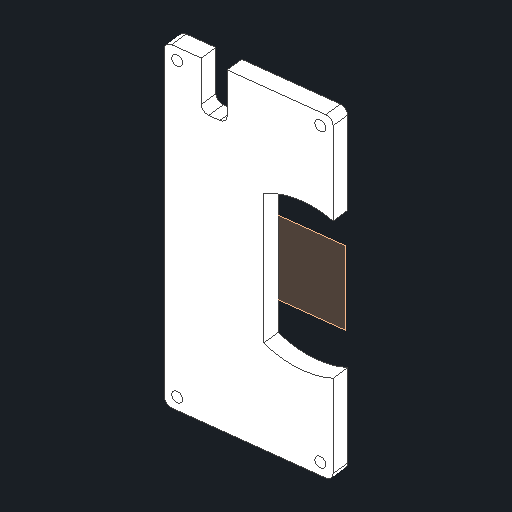
# Autodesk Inventor part: TAPA_CAMARA_2
Saved by Autodesk Inventor 2024.3 (Build 283343000, 343)
## iProperties
Created: 2024-07-21
Part Number: TAPA_CAMARA_2
Material: Generic
Document SubType Name: Modeling
Designer: Niler
Density: 1 g/cm^3
Appearance: Default
Author: Niler
Autodesk Inventor part; units mm, degrees
ref_plane "YZ Plane" through (0, 0, 0) normal (1, 0, 0) x (0, 1, 0)
ref_plane "XZ Plane" through (0, 0, 0) normal (0, 1, 0) x (-1, 0, 0)
ref_plane "XY Plane" through (0, 0, 0) normal (0, 0, 1) x (1, 0, 0)
ref_plane "Work Plane1" through (-27.4782, 47.3, -1.2107) normal (0.118263, 0, 0.9929823) x (0, -1, 0)
sketch "Sketch1" plane through (-27.4782, 47.3, -1.2107) normal (0.118263, 0, 0.9929823) x (0, -1, 0)
  line L0 (0, 33.4421) -> (0, -8.2516) projected
  line L1 (2, -10.2376) -> (92.6, -10.2376) projected
  line L2 (94.6, -8.2516) -> (94.6, 33.4421) projected
  line L3 (92.6, 35.428) -> (2, 35.428) projected
  line L4 (7, -3.2867) -> (7, 28.4771) projected
  line L5 (7, 28.4771) -> (87.6, 28.4771) projected
  line L6 (87.6, 28.4771) -> (87.6, -3.2867) projected
  line L7 (87.6, -3.2867) -> (7, -3.2867) projected
  ellipse E0 centre (2, 33.4421) end of major axis (4, 33.4421) minor radius 1.986 (2, 35.428) -> (0, 33.4421) ccw projected
  ellipse E1 centre (2, -8.2516) end of major axis (0, -8.2516) minor radius 1.986 (0, -8.2516) -> (2, -10.2376) ccw projected
  ellipse E2 centre (92.6, -8.2516) end of major axis (90.6, -8.2516) minor radius 1.986 (92.6, -10.2376) -> (94.6, -8.2516) ccw projected
  ellipse E3 centre (92.6, 33.4421) end of major axis (94.6, 33.4421) minor radius 1.986 (94.6, 33.4421) -> (92.6, 35.428) ccw projected
  ellipse E4 centre (91.1, -6.7621) end of major axis (92.6, -6.7621) minor radius 1.4895 projected
  ellipse E5 centre (3.5, -6.7621) end of major axis (5, -6.7621) minor radius 1.4895 projected
  ellipse E6 centre (91.1, 31.9526) end of major axis (92.6, 31.9526) minor radius 1.4895 projected
  ellipse E7 centre (3.5, 31.9526) end of major axis (5, 31.9526) minor radius 1.4895 projected
  point P0 (47.3, 27.1422)
  constraints: 4 other
extrude "Extrusion1" add sketch "Sketch1" along normal blind 5 contours E0 L3 E3 L2 E2 L1 E1 L0 | L4 L5 L6 L7
sketch "Sketch2" plane through (-26.8869, 47.3, 3.7542) normal (0.118263, 0, 0.9929823) x (0.9929823, 0, -0.118263)
  line L0 (16.6422, -25.3) -> (37.6422, -25.3)
  line L1 (37.6422, -25.3) -> (37.6422, -69.3)
  line L2 (37.6422, -69.3) -> (16.6422, -69.3)
  line L3 (16.6422, -69.3) -> (16.6422, -25.3)
  line L4 (16.6422, -25.3) -> (37.6422, -69.3) construction
  line L5 (37.6422, -25.3) -> (16.6422, -69.3) construction
  line L6 (37.6422, -27.8) -> (16.6422, -27.8)
  arc A0 (37.6422, -27.8) -> (16.6422, -27.8) centre (27.1422, -48.6) ccw
  line L7 (33.4421, 0) -> (-8.2516, 0) projected
  arc A1 (-8.2516, 0) -> (-10.2376, -2) centre (2, -2) ccw projected
  line L8 (-10.2376, -2) -> (-10.2376, -92.6) projected
  arc A2 (-10.2376, -92.6) -> (-8.2516, -94.6) centre (2, -92.6) ccw projected
  line L9 (-8.2516, -94.6) -> (33.4421, -94.6) projected
  arc A3 (33.4421, -94.6) -> (35.428, -92.6) centre (45.9099, -92.6) ccw projected
  line L10 (35.428, -92.6) -> (35.428, -2) projected
  arc A4 (35.428, -2) -> (33.4421, 0) centre (45.9099, -2) ccw projected
  circle A5 centre (44.4099, -3.5) radius 1.5 projected
  circle A6 centre (44.4099, -91.1) radius 1.5 projected
  circle A7 centre (3.5, -3.5) radius 1.5 projected
  circle A8 centre (3.5, -91.1) radius 1.5 projected
  line L11 (35.428, -47.3) -> (-10.2376, -47.3)
  line L12 (-10.2376, -2) -> (-10.2376, -92.6) projected
  arc A9 (16.6422, -66.8) -> (37.6422, -66.8) centre (27.1422, -46) ccw
  point P0 (27.1422, -47.3)
  point P1 (27.1422, -25.3)
  point P2 (16.6422, -66.8)
  point P3 (37.6422, -66.8)
  dimension "d2" = 21
  dimension "d3" = 44
  dimension "d4" = 2.5
  constraints: 16 end point, 5 midpoint, 5 point on circle, 3 symmetric about line, 2 centre point, 2 parallel, 2 perpendicular, 2 point on line, 1 horizontal, 5 other
  measures "d2" distance of L1.end L2.end
  measures "d3" distance of L0.end L1.end
  measures "d4" distance between parallel lines of L0 L6
extrude "Extrusion2" cut sketch "Sketch2" against normal through all contours A0 L10 L6 | L6 L10 L11 L3 | A0 L6 L10 | L11 L10 A9 L3 | L6 L1 A9 L10
sketch "Sketch3" plane through (-27.4782, 47.3, -1.2107) normal (-0.118263, 0, -0.9929823) x (-0.9929823, 0, 0.118263)
  arc A0 (-35.428, -67.7769) -> (-16.6422, -66.8) centre (-27.1422, -46) ccw projected
  arc A1 (-16.6422, -27.8) -> (-35.428, -26.8231) centre (-27.1422, -48.6) ccw projected
  line L0 (-16.6422, -27.8) -> (-16.6422, -66.8) projected
  line L1 (-33.4421, 0) -> (8.2516, 0) projected
  arc A2 (-33.4421, 0) -> (-35.428, -2) centre (-45.9099, -2) ccw projected
  line L2 (-35.428, -92.6) -> (-35.428, -67.7769) projected
  arc A3 (-35.428, -92.6) -> (-33.4421, -94.6) centre (-45.9099, -92.6) ccw projected
  line L3 (8.2516, -94.6) -> (-33.4421, -94.6) projected
  arc A4 (8.2516, -94.6) -> (10.2376, -92.6) centre (-2, -92.6) ccw projected
  line L4 (10.2376, -2) -> (10.2376, -92.6) projected
  arc A5 (10.2376, -2) -> (8.2516, 0) centre (-2, -2) ccw projected
  circle A6 centre (-44.4099, -3.5) radius 1.5 projected
  circle A7 centre (-44.4099, -91.1) radius 1.5 projected
  circle A8 centre (-3.5, -3.5) radius 1.5 projected
  circle A9 centre (-3.5, -91.1) radius 1.5 projected
  line L5 (-6.7624, 0) -> (0.2376, 0)
  line L6 (0.2376, 0) -> (0.2376, -12.0472)
  line L7 (-1.7624, -14.0472) -> (-4.7624, -14.0472)
  line L8 (-6.7624, -12.0472) -> (-6.7624, 0)
  arc A10 (-6.7624, -12.0472) -> (-4.7624, -14.0472) centre (-4.7624, -12.0472) ccw
  arc A11 (-1.7624, -14.0472) -> (0.2376, -12.0472) centre (-1.7624, -12.0472) ccw
  line L9 (0.2376, -7) -> (-6.7624, -7)
  line L10 (-35.428, -26.8231) -> (-35.428, -2) projected
  point P0 (-27.1422, -47.3)
  point P1 (0.2376, -14.0472)
  point P2 (-6.7624, -14.0472)
  point P3 (0.2376, 0)
  dimension "d7" = 7
  dimension "d9" = 2
  dimension "d12" = 10
  dimension "d13" = 7
  constraints: 10 end point, 7 point on line, 4 point on circle, 4 tangent, 2 centre point, 2 parallel, 2 perpendicular, 1 equal radius, 1 horizontal, 4 other
  measures "d7" distance of point (0.238, -14.047) point (-6.762, -14.047)
  measures "d9" radius of A10
  measures "d12" distance between parallel lines of L4 L6
  measures "d13" distance between parallel lines of L1 L9
extrude "Extrusion3" cut sketch "Sketch3" against normal through all contours L1 L6 L9 L8 | L9 L6 A11 L7 A10 L8 | A8
body "Solid1"
